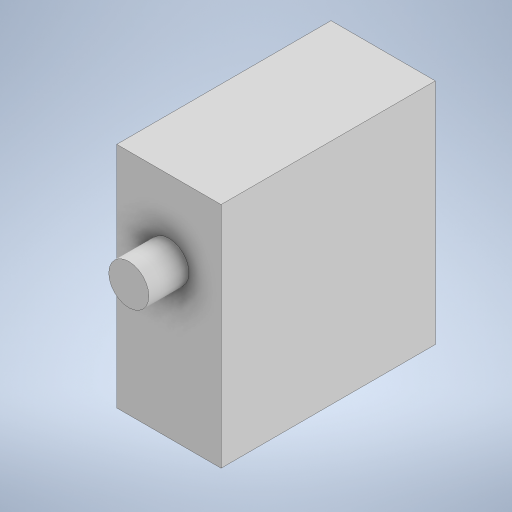
# Autodesk Inventor part: servoRep
Saved by Autodesk Inventor 2024.3 (Build 283343000, 343)
## iProperties
Created: 2025-01-11
Part Number: servoRep
Material: Generic
Document SubType Name: Modeling
Designer: jjrwe
Density: 1 g/cm^3
Appearance: Default
Author: jjrwe
Autodesk Inventor part; units mm, degrees
ref_plane "YZ Plane" through (0, 0, 0) normal (1, 0, 0) x (0, 1, 0)
ref_plane "XZ Plane" through (0, 0, 0) normal (0, 1, 0) x (-1, 0, 0)
ref_plane "XY Plane" through (0, 0, 0) normal (0, 0, 1) x (1, 0, 0)
sketch "Sketch1" plane through (0, 0, 0) normal (0, 0, 1) x (1, 0, 0)
  line L0 (0, 0) -> (13, 0)
  line L1 (13, 0) -> (13, 28.45)
  line L2 (13, 28.45) -> (0, 28.45)
  line L3 (0, 28.45) -> (0, 0)
  dimension "d0" = 13
  dimension "d1" = 28.45
  constraints: 8 end point, 2 parallel, 1 horizontal, 1 perpendicular
  measures "d0" distance of L2.end L1.end
  measures "d1" distance of L1.end L0.end
extrude "Extrusion1" add sketch "Sketch1" along normal blind 26.7
sketch "Sketch2" plane through (0, 0, 26.7) normal (0, 0, 1) x (1, 0, 0)
  line L0 (13, 28.45) -> (0, 28.45) projected
  circle A0 centre (6.5, 19.07) radius 2.5
  point P0 (0, 0)
  dimension "d5" = 5
  constraints: 1 centre point
  measures "d5" diameter of A0
extrude "Extrusion2" add sketch "Sketch2" along normal blind 5
body "Solid1"
